test nub (Autodesk Fusion 360 design; units mm, degrees)
Autodesk Fusion 360 part; units mm, degrees
sketch "Sketch1" plane through (0, 0, 0) normal (0, 0, 1) x (1, 0, 0)
  line L0 (-7.9259, 8.6629) -> (-2.1165, 8.6629)
  line L1 (-1.5, 1) -> (-1.5, -1)
  line L2 (-2.1165, -8.6629) -> (-7.9259, -8.6629)
  line L3 (-7.9259, -8.6629) -> (-7.9259, 8.6629)
  line L4 (2.1165, 8.6629) -> (7.9259, 8.6629)
  line L5 (7.9259, 8.6629) -> (7.9259, -8.6629)
  line L6 (7.9259, -8.6629) -> (2.11, -8.6629)
  line L7 (1.5, -1) -> (1.5, 1)
  line L8 (-48.0743, 0) -> (41.8844, 0) construction
  line L9 (1.5, 18.5935) -> (0, 18.5935) construction
  line L10 (0, 0) -> (0, 17.2446) construction
  line L11 (0, 18.5935) -> (-1.5, 18.5935) construction
  line L12 (-1.5, 1) -> (1.5, 1)
  line L13 (1.5, 1) -> (1.5, -1)
  line L14 (1.5, -1) -> (-1.5, -1)
  line L15 (-1.5, -1) -> (-1.5, 1)
  line L16 (-2.1165, 8.6629) -> (-1.5, 1)
  line L17 (-1.5, -1) -> (-2.1165, -8.6629)
  line L18 (2.11, -8.6629) -> (1.5, -1)
  line L19 (-1.5, -1) -> (-1.5, -18.4253) construction
  line L20 (1.5, 0) -> (7.9259, 0) construction
  line L21 (-1.5, 0) -> (-7.9259, 0) construction
  line L22 (1.5, 1) -> (2.1165, 8.6629)
  line L23 (-1.5, 1) -> (-1.5, 16.5395) construction
  point P0 (1.5, 0)
  point P1 (-1.5, 0)
  point P2 (1.5, 0)
  point P3 (7.9259, 0)
  point P4 (-7.9259, 0)
  dimension "d1" = 4.6
  dimension "d2" = 4.6
  dimension "d3" = 2
  dimension "d8" = 3
  constraint horizontal L0
  constraint vertical L1
  constraint horizontal L2
  constraint vertical L3
  constraint horizontal L4
  constraint vertical L5
  constraint horizontal L6
  constraint vertical L7
  constraint perpendicular L1 L8
  constraint coincident L10.start L8
  constraint coincident L8 P2
  constraint coincident L8 P1
  constraint coincident L7 L9.start
  constraint coincident L1 L11.end
  constraint perpendicular L1 L9
  constraint coincident L10.start origin
  constraint perpendicular L8 L10
  constraint coincident L10 L9.end
  constraint perpendicular L1 L11
  constraint equal L9 L11
  constraint horizontal L12
  constraint horizontal L14
  constraint vertical L15
  constraint midpoint L13 P2
  constraint coincident L7 P2
  constraint coincident L1 P1
  constraint perpendicular L14 L19
  constraint equal L0 L4
  constraint coincident P2 P0
  constraint coincident L5 P3
  constraint coincident L8 P3
  constraint coincident P1 L21.start
  constraint coincident L8 P4
  constraint coincident L3 P4
  constraint equal L20 L21
  constraint perpendicular L12 L23
  constraint equal L3 L5
  constraint midpoint L5 P3
  constraint midpoint L3 P4
  measures "d1" angle of L17 L19
  measures "d2" angle of L16 L23
  measures "d3" distance of L12 L14
  measures "d8" distance of L7.start L1.end
extrude "Extrude1" add sketch "Sketch1" along normal blind 14
fillet "Fillet1" radius 1 4 edges at (-1.5, -1, 7) (1.5, -1, 7) (-1.5, 1, 7) (1.5, 1, 7)
equation "d2 = d1"
